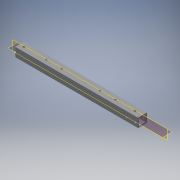
# Autodesk Inventor part: Large crossbeam
Saved by Autodesk Inventor 2017 (Build 210142000, 142)
## iProperties
Created: 2016-09-25
Part Number: Large crossbeam
Material: Generic
Document SubType Name: Sheet Metal
Designer: Hanson
Density: 1 g/cm^3
Sheet Metal Rule: Default
Appearance: Default
Author: Hanson
Autodesk Inventor part; units mm, degrees
ref_plane "YZ Plane" through (0, 0, 0) normal (1, 0, 0) x (0, 1, 0)
ref_plane "XZ Plane" through (0, 0, 0) normal (0, 1, 0) x (-1, 0, 0)
ref_plane "XY Plane" through (0, 0, 0) normal (0, 0, 1) x (1, 0, 0)
sketch "Sketch1" plane through (0, 0, 0) normal (0, 1, 0) x (-1, 0, 0)
  line L0 (0, 0) -> (-349.25, 0)
  line L1 (-349.25, 0) -> (-349.25, -25.4)
  line L2 (-349.25, -25.4) -> (0, -25.4)
  line L3 (0, -25.4) -> (0, 0)
  dimension "d0" = 349.25
  dimension "d1" = 25.4
  constraints: 8 end point, 2 parallel, 1 horizontal, 1 perpendicular
  measures "d0" distance of L2.end L1.end
  measures "d1" distance of L0.end L1.end
extrude "Extrusion1" add sketch "Sketch1" along normal blind 3.175
sketch "Sketch2" plane through (0, 3.175, 0) normal (0, 1, 0) x (1, 0, 0)
  line L0 (349.25, 25.4) -> (0, 25.4) projected
  line L1 (0, 25.4) -> (0, 0) projected
  point P0 (12.7, 12.7)
  dimension "d4" = 12.7
  dimension "d5" = 12.7
  measures "d4" distance from line of L0 point (12.7, 12.7)
  measures "d5" distance from line of L1 point (12.7, 12.7)
hole "Hole1" at (12.7, 3.175, -12.7) direction (0, -1, 0) diameter 6.35 end through all
sketch "Sketch3" plane through (0, 3.175, 0) normal (0, 1, 0) x (1, 0, 0)
  line L0 (0, 25.4) -> (0, 0) projected
  line L1 (349.25, 25.4) -> (0, 25.4) projected
  point P0 (76.2, 12.7)
  point P1 (228.854, 12.7)
  dimension "d13" = 76.2
  dimension "d14" = 12.7
  dimension "d106" = 12.7
  dimension "d107" = 152.654
  measures "d13" distance from line of L0 point (76.2, 12.7)
  measures "d14" distance from line of L1 point (76.2, 12.7)
  measures "d106" distance from line of L1 point (228.854, 12.7)
  measures "d107" distance of point (76.2, 12.7) point (228.854, 12.7)
hole "Hole2" at (76.2, 3.175, -12.7) at (228.854, 3.175, -12.7) direction (0, -1, 0) diameter 5.1562 end through all
ref_plane "Work Plane1" through (174.625, 0, 0) normal (1, 0, 0) x (0, 0, -1)
mirror "Mirror1" about plane through (174.625, 0, 0) normal (1, 0, 0) of "Hole2", "Hole1"
sketch "Sketch7" plane through (0, 3.175, 0) normal (0, 1, 0) x (1, 0, 0)
  line L0 (349.25, 0) -> (349.25, 25.4) projected
  line L1 (0, 0) -> (349.25, 0)
  line L2 (349.25, 0) -> (349.25, 3.175)
  line L3 (349.25, 3.175) -> (0, 3.175)
  line L4 (0, 3.175) -> (0, 0)
  dimension "d49" = 3.175
  constraints: 8 end point, 2 parallel, 1 horizontal, 1 perpendicular, 1 point on line
  measures "d49" distance of L2.end L1.end
extrude "Extrusion2" add sketch "Sketch7" along normal blind 22.225
ref_plane "Work Plane2" through (0, 0, -12.7) normal (0, 0, 1) x (1, 0, 0)
mirror "Mirror2" about plane through (0, 0, -12.7) normal (0, 0, 1) of "Extrusion2"
sketch "Sketch8" plane through (0, 3.175, -22.225) normal (0, 0, 1) x (1, 0, 0)
  line L0 (349.25, 22.225) -> (0, 22.225) projected
  line L1 (349.25, 22.225) -> (0, 22.225)
  line L2 (0, 22.225) -> (0, 19.05)
  line L3 (0, 19.05) -> (349.25, 19.05)
  line L4 (349.25, 19.05) -> (349.25, 22.225)
  point P0 (0, -3.175)
  dimension "d52" = 349.25
  dimension "d53" = 3.175
  constraints: 8 end point, 2 parallel, 1 horizontal, 1 perpendicular
  measures "d52" distance of L3.end L2.end
  measures "d53" distance of L2.end L1.end
extrude "Extrusion3" add sketch "Sketch8" along normal blind 19.05
ref_plane "Work Plane3" through (0, 12.7, 0) normal (0, -1, 0) x (1, 0, 0)
mirror "Mirror3" about plane through (0, 12.7, 0) normal (0, -1, 0) of "Hole2", "Hole1", "Mirror1"
sketch "Sketch10" plane through (349.25, 0, -25.4) normal (0, 0, -1) x (-1, 0, 0)
  line L0 (0, 0) -> (349.25, 0) projected
  line L1 (0, 0) -> (0, 25.4) projected
  point P0 (33.6956, 10.1854)
  dimension "d61" = 10.1854
  dimension "d62" = 33.6956
  measures "d61" distance from line of L0 point (33.696, 10.185)
  measures "d62" distance from line of L1 point (33.696, 10.185)
sketch "Sketch11" plane through (349.25, 0, -25.4) normal (0, 0, -1) x (-1, 0, 0)
  line L0 (0, 0) -> (349.25, 0) projected
  line L1 (0, 0) -> (0, 25.4) projected
  point P0 (8.2956, 10.1854)
  dimension "d70" = 10.1854
  dimension "d71" = 8.2956
  measures "d70" distance from line of L0 point (8.296, 10.185)
  measures "d71" distance from line of L1 point (8.296, 10.185)
hole "Hole8" at (315.5544, 10.1854, -25.4) direction (0, 0, 1) diameter 5.1594 end through all
hole "Hole9" at (340.9544, 10.1854, -25.4) direction (0, 0, 1) diameter 5.1594 end through all
sketch "Sketch12" plane through (0, 12.7, 0) normal (0, -1, 0) x (1, 0, 0)
  point P0 (0, 0)
sketch "Sketch13" plane through (0, 0, 0) normal (0, -1, 0) x (1, 0, 0)
  line L0 (349.25, 0) -> (349.25, -25.4) projected
  line L1 (349.25, -25.4) -> (0, -25.4) projected
  circle A0 centre (336.55, -12.7) radius 3.175
  point P0 (0, 0)
  dimension "d93" = 12.7
  dimension "d94" = 12.7
  constraints: 1 centre point, 1 coincident
  measures "d93" distance from line of L0 point (336.55, -12.7)
  measures "d94" distance from line of L1 point (336.55, -12.7)
extrude "Extrusion5" add sketch "Sketch13" against normal blind 3.175
mirror "Mirror4" about plane through (0, 12.7, 0) normal (0, -1, 0) of "Extrusion5"
sketch "Sketch14" plane through (0, 0, 0) normal (0, -1, 0) x (1, 0, 0)
  line L0 (349.25, 0) -> (349.25, -25.4) projected
  line L1 (349.25, -25.4) -> (0, -25.4) projected
  point P0 (0, 0)
  point P1 (328.2442, -12.7)
  dimension "d97" = 21.0058
  dimension "d98" = 12.7
  measures "d97" distance from line of L0 point (328.244, -12.7)
  measures "d98" distance from line of L1 point (328.244, -12.7)
hole "Hole10" at (328.2442, 0, -12.7) direction (0, 1, 0) diameter 6.35 end through all
equation "\"d11\" = Thickness"
equation "\"d20\" = Thickness"
equation "\"d84\" = Thickness"
equation "\"d91\" = Thickness"
equation "\"d104\" = Thickness"
equation "\"BendRadius\" = Thickness"
equation "\"BendReliefWidth\" = Thickness"
equation "\"BendReliefDepth\" = 0.5 * Thickness"
equation "\"CornerReliefSize\" = 4 * Thickness"
equation "\"MinimumRemnant\" = 2 * Thickness"
equation "\"TransitionRadius\" = BendRadius"
equation "\"JacobiRadiusSize\" = BendRadius"
equation "\"GapSize\" = Thickness"
equation "\"Thickness\" = 3.048"
body "Solid1"
